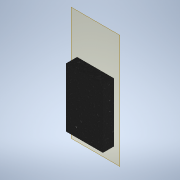
# Autodesk Inventor part: rubber padding
Saved by Autodesk Inventor 2020 (Build 240168000, 168)
## iProperties
Created: 2020-07-02
Part Number: rubber padding
Material: Generic
Document SubType Name: Modeling
Designer: Ashiqrahman
Density: 1 g/cm^3
Appearance: Fine Textured - Black
Author: Ashiqrahman
Autodesk Inventor part; units mm, degrees
ref_plane "YZ Plane" through (0, 0, 0) normal (1, 0, 0) x (0, 1, 0)
ref_plane "XZ Plane" through (0, 0, 0) normal (0, 1, 0) x (-1, 0, 0)
ref_plane "XY Plane" through (0, 0, 0) normal (0, 0, 1) x (1, 0, 0)
ref_plane "Work Plane1" through (-136.8843, -40.4621, -113.009) normal (0, 0, 1) x (1, 0, 0)
sketch "Sketch1" plane through (-136.8843, -40.4621, -113.009) normal (0, 0, 1) x (1, 0, 0)
  line L0 (-25, -40) -> (25, -40)
  line L1 (25, -40) -> (25, 40)
  line L2 (25, 40) -> (-25, 40)
  line L3 (-25, 40) -> (-25, -40)
  line L4 (-25, -40) -> (25, 40) construction
  line L5 (25, -40) -> (-25, 40) construction
  point P0 (136.8843, 40.4621)
  point P1 (0, 0)
  dimension "d0" = 50
  dimension "d1" = 80
  constraints: 12 end point, 2 midpoint, 2 parallel, 1 horizontal, 1 perpendicular
  measures "d0" distance of L2.end L1.end
  measures "d1" distance of L1.end L0.end
extrude "Extrusion1" add sketch "Sketch1" along normal blind 15
fillet "Fillet1" radius 8 4 edges at (-136.8843, -80.4621, -98.009) (-111.8843, -40.4621, -98.009) (-136.8843, -0.4621, -98.009) (-161.8843, -40.4621, -98.009)
body "Solid1"
